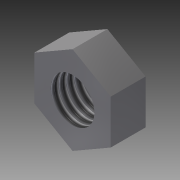
# Autodesk Inventor part: M4Nut
Saved by Autodesk Inventor 2015 SP1 (Build 190203100, 203)
## iProperties
Company: Misumi
Category: Hardware
Created: 2013-12-08
Part Number: M4Nut
Material: Steel, Alloy
Document SubType Name: Modeling
Designer: Jack
Density: 7.73 g/cm^3
Appearance: Semi-Polished
Mass: 0.738836 g
Surface Area: 1.77546 cm^2
Volume: 0.0955804 cm^3
Vendor: Misumi
Catalog Web Link: http://us.misumi-ec.com/vona2/detail/110300250540/
Stock Number: KNTR4
Author: Jack
Title: M4 Nut
Autodesk Inventor part; units mm, degrees
ref_plane "YZ Plane" through (0, 0, 0) normal (1, 0, 0) x (0, 1, 0)
ref_plane "XZ Plane" through (0, 0, 0) normal (0, 1, 0) x (-1, 0, 0)
ref_plane "XY Plane" through (0, 0, 0) normal (0, 0, 1) x (1, 0, 0)
sketch "Sketch1" plane through (0, 0, 0) normal (0, 1, 0) x (-1, 0, 0)
  line L0 (0, 4.0415) -> (3.5, 2.0207)
  line L1 (3.5, 2.0207) -> (3.5, -2.0207)
  line L2 (3.5, -2.0207) -> (0, -4.0415)
  line L3 (0, -4.0415) -> (-3.5, -2.0207)
  line L4 (-3.5, -2.0207) -> (-3.5, 2.0207)
  line L5 (-3.5, 2.0207) -> (0, 4.0415)
  point P0 (0, 0)
  point P1 (0, 0)
  dimension "d0" = 3.5
  constraints: 12 end point, 1 coincident, 1 vertical, 13 other
  measures "d0" distance from line of point (0, 0) L4
extrude "Extrusion1" add sketch "Sketch1" along normal blind 3.2
sketch "Sketch2" plane through (0, 3.2, 0) normal (0, 1, 0) x (1, 0, 0)
  circle A0 centre (0, 0) radius 2
  dimension "d3" = 4
  constraints: 1 centre point, 1 coincident
  measures "d3" diameter of A0
extrude "Extrusion2" cut sketch "Sketch2" against normal blind 4.3
thread "Thread1" size "M4x0.7" class "6H" standard "ANSI Metric M Profile" full length
body "Solid1"
